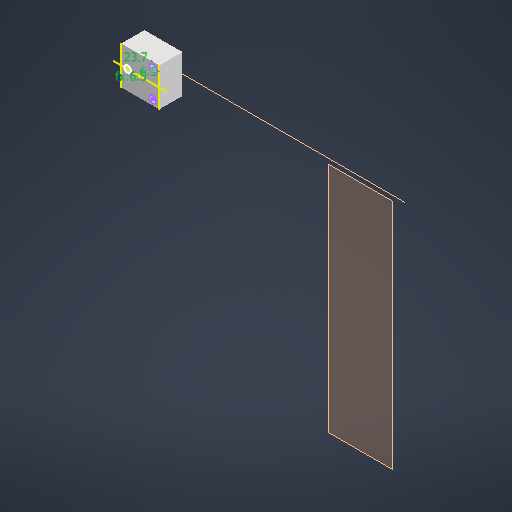
# Autodesk Inventor part: Camera_mount
Saved by Autodesk Inventor 2027.1 (Build 311270010, 270A)
## iProperties
Created: 2026-09-16
Part Number: Camera_mount
Material: Generic
Document SubType Name: Modeling
Designer: Jacob Parker
Density: 1 g/cm^3
Appearance: Default
Author: Jacob Parker
Autodesk Inventor part; units mm, degrees
ref_plane "YZ Plane" through (0, 0, 0) normal (1, 0, 0) x (0, 1, 0)
ref_plane "XZ Plane" through (0, 0, 0) normal (0, 1, 0) x (-1, 0, 0)
ref_plane "XY Plane" through (0, 0, 0) normal (0, 0, 1) x (1, 0, 0)
ref_plane "Work Plane1" through (186.7197, -114.7807, 0) normal (0, 0, 1) x (1, 0, 0)
sketch "Sketch1" plane through (186.7197, -114.7807, 0) normal (0, 0, 1) x (1, 0, 0)
  line L0 (-168.7197, 132.7807) -> (-204.7197, 132.7807)
  line L1 (-204.7197, 132.7807) -> (-204.7197, 96.7807)
  line L2 (-204.7197, 96.7807) -> (-168.7197, 96.7807)
  line L3 (-168.7197, 96.7807) -> (-168.7197, 132.7807)
  point P0 (-186.7197, 114.7807)
  point P1 (-168.7197, 114.7807)
  point P2 (-186.7197, 96.7807)
  point P3 (-204.7197, 114.7807)
  dimension "d0" = 36
  dimension "d1" = 36
  dimension "d8" = 0
  dimension "d9" = 0
  constraints: 8 end point, 3 midpoint, 2 parallel, 1 horizontal, 1 perpendicular
  measures "d0" distance of L2.end L0.start
  measures "d1" distance of L1.end L2.end
  measures "d8" horizontal distance of point (-186.72, 114.781) point (-186.72, 96.781)
  measures "d9" vertical distance of point (-186.72, 114.781) point (-204.72, 114.781)
extrude "Extrusion1" add sketch "Sketch1" along normal blind 22
sketch "Sketch3" plane through (186.7197, -114.7807, 22) normal (0, 0, 1) x (1, 0, 0)
  circle A0 centre (-174.8697, 127.7151) radius 3.25
  circle A1 centre (-198.5697, 114.7807) radius 3.25
  line L0 (-211.9197, 114.7807) -> (-161.5197, 114.7807) projected
  circle A2 centre (-174.8697, 101.8464) radius 3.25
  line L1 (-174.8697, 127.7151) -> (-168.7197, 127.7151)
  line L2 (-168.7197, 96.7807) -> (-168.7197, 132.7807) projected
  line L3 (-198.5697, 114.7807) -> (-204.7197, 114.7807)
  line L4 (-204.7197, 132.7807) -> (-204.7197, 96.7807) projected
  point P0 (-186.7197, 114.7807)
  dimension "d10" = 6.5
  dimension "d11" = 6.5
  dimension "d12" = 23.7
  constraints: 4 end point, 3 centre point, 2 point on line, 1 horizontal, 1 midpoint, 1 parallel, 1 symmetric about line, 1 other
  measures "d10" diameter of A0
  measures "d11" diameter of A1
  measures "d12" horizontal distance of L1.start L3.start
hole "Hole1" at (11.85, -12.9344, 22) at (11.85, 12.9344, 22) at (-11.85, 0, 22) direction (0, 0, -1) diameter 6.5 depth 6
hole "Hole2" at (-11.85, 0, 22) at (11.85, -12.9344, 22) at (11.85, 12.9344, 22) direction (0, 0, -1) diameter 4 end through all
equation "\"d1\" = d0"
equation "\"d11\" = d10"
body "Solid1"
